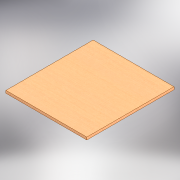
# Autodesk Inventor part: wooden_base
Saved by Autodesk Inventor 2020 (Build 240168000, 168)
## iProperties
Created: 2020-06-18
Part Number: wooden_base
Material: Generic
Document SubType Name: Modeling
Designer: pc-konvi
Density: 1 g/cm^3
Appearance: Cherry - Natural Low Gloss
Author: pc-konvi
Autodesk Inventor part; units mm, degrees
ref_plane "YZ Plane" through (0, 0, 0) normal (1, 0, 0) x (0, 1, 0)
ref_plane "XZ Plane" through (0, 0, 0) normal (0, 1, 0) x (-1, 0, 0)
ref_plane "XY Plane" through (0, 0, 0) normal (0, 0, 1) x (1, 0, 0)
sketch "Sketch1" plane through (0, 0, 0) normal (0, 1, 0) x (-1, 0, 0)
  line L0 (-160, -172.5) -> (160, -172.5)
  line L1 (160, -172.5) -> (160, 172.5)
  line L2 (160, 172.5) -> (-160, 172.5)
  line L3 (-160, 172.5) -> (-160, -172.5)
  line L4 (-160, -172.5) -> (160, 172.5) construction
  line L5 (160, -172.5) -> (-160, 172.5) construction
  point P0 (0, 0)
  dimension "d0" = 345
  dimension "d1" = 320
  constraints: 12 end point, 2 midpoint, 2 parallel, 1 horizontal, 1 perpendicular
  measures "d0" distance of L0.end L1.end
  measures "d1" distance of L1.end L2.end
extrude "Extrusion1" add sketch "Sketch1" along normal blind 10
body "Solid1"
